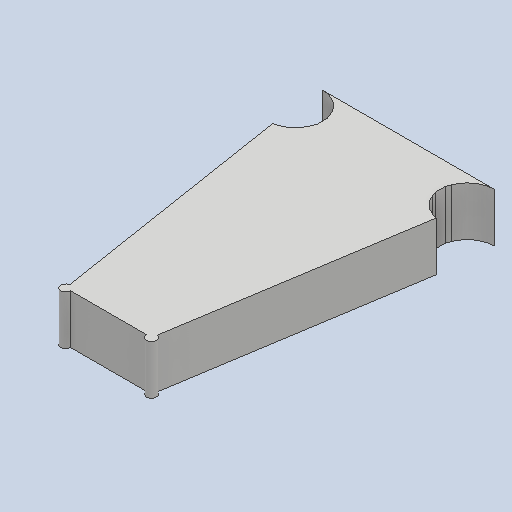
# Autodesk Inventor part: ч ASY human dummy 01
Saved by Autodesk Inventor 2025 (Build 290162010, 162A)
## iProperties
Created: 2018-05-28
Part Number: ч ASY human dummy 01
Material: Типовые
Document SubType Name: Modeling
Designer: admin
Density: 1 g/cm^3
Appearance: По умолчанию
Author: admin
Autodesk Inventor part; units mm, degrees
ref_plane "YZ Plane" through (0, 0, 0) normal (1, 0, 0) x (0, 1, 0)
ref_plane "XZ Plane" through (0, 0, 0) normal (0, 1, 0) x (-1, 0, 0)
ref_plane "XY Plane" through (0, 0, 0) normal (0, 0, 1) x (1, 0, 0)
sketch "Эскиз1" plane through (0, 0, 0) normal (0, 0, 1) x (1, 0, 0)
  line L0 (-175, 0) -> (175, 0)
  line L1 (0, 0) -> (0, -465)
  line L2 (0, -465) -> (-87.5, -555)
  line L3 (-87.5, -555) -> (87.5, -555)
  line L4 (87.5, -555) -> (0, -465)
  circle A0 centre (175, 0) radius 55
  circle A1 centre (-175, 0) radius 55
  circle A2 centre (87.5, -555) radius 70
  circle A3 centre (-87.5, -555) radius 70
  line L5 (175, 0) -> (87.5, -555)
  line L6 (-175, 0) -> (-87.5, -555)
  line L7 (175, 55) -> (-175, 55)
  line L8 (87.5, -625) -> (-87.5, -625)
  line L9 (-120, 10) -> (-120, -10)
  line L10 (120, 10) -> (120, -10)
  line L11 (-120, 10) -> (-123.52, 19.36)
  line L12 (-120, -10) -> (-123.52, -19.36)
  line L13 (120, 10) -> (123.52, 19.36)
  line L14 (120, -10) -> (123.52, -19.36)
  circle A4 centre (87.5, -555) radius 10
  circle A5 centre (-87.5, -555) radius 10
  point P0 (0, -555)
  point P1 (166.4346, -54.3289)
  point P2 (-166.4346, -54.3289)
  point P3 (-98.4014, -485.8541)
  point P4 (98.4014, -485.8541)
  point P5 (120, 0)
  point P6 (-120, 0)
  point P7 (-38.7045, -504.8104)
  point P8 (38.7045, -504.8104)
  point P9 (89.0573, -545.122)
  point P10 (-89.0573, -545.122)
  point P11 (-77.5, -555)
  point P12 (77.5, -555)
  dimension "d10" = 140
  dimension "d11" = 140
  dimension "d4" = 90
  dimension "d5" = 175
  dimension "d6" = 350
  dimension "d7" = 110
  dimension "d8" = 110
  dimension "d9" = 465
  dimension "d14" = 20
  dimension "d15" = 20
  dimension "d16" = 20
  dimension "d17" = 20
  constraints: 30 end point, 8 tangent, 7 coincident, 6 point on circle, 4 centre point, 4 horizontal, 4 midpoint, 2 horizontal alignment, 2 perpendicular, 2 vertical, 1 vertical alignment, 6 other
  measures "d4" distance from line of L1.end L3
  measures "d5" distance of L2.end L3.end
  measures "d6" distance of L0.start L0.end
  measures "d7" diameter of A1
  measures "d8" diameter of A0
  measures "d9" distance of L1.start L1.end
  measures "d14" distance of L9.start L9.end
  measures "d15" distance of L10.start L10.end
  measures "d16" diameter of A4
  measures "d17" diameter of A5
extrude "Выдавливание1" add sketch "Эскиз1" along normal mid plane 100 contours L9 L11 A1 L7 A0 L13 L10 L0 | L0 L1 L2 A3 L6 A1 L12 L9 | L0 L10 L14 A0 L5 A2 L4 L1 | A3 L2 A5 L6 | L4 A2 L3 A3 L2 | A3 L3 A5 L2 | A5 L2 L6 | L6 L3 A5 | A2 L5 A4 L4 | L4 A4 L3 A2 | A5 L3 L2 | A4 L5 L4 | L4 L3 A4 | L5 A4 L3
equation "\"d10\" = hip_diam"
equation "\"d11\" = d10"
equation "\"d4\" = hip_joint_hight"
equation "\"d5\" = hip_joint_width"
equation "\"d6\" = clavicular_width"
equation "\"d7\" = shoulder_radius"
equation "\"d8\" = d7"
equation "\"hip_diam\" = 140"
equation "\"hip_joint_hight\" = 90"
equation "\"hip_joint_width\" = 175"
equation "\"clavicular_width\" = 350"
equation "\"shoulder_radius\" = 110"
